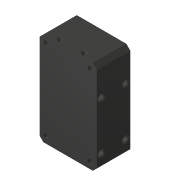
# Autodesk Inventor part: XM430_HOUSING_MIDDLE
Saved by Autodesk Inventor 2019.4 (Build 234330000, 330)
## iProperties
Created: 2019-10-08
Part Number: XM430_HOUSING_MIDDLE
Material: 一般
Document SubType Name: Modeling
Designer: y6tada
Density: 1 g/cm^3
Appearance: 滑らか - 黒
Author: y6tada
Autodesk Inventor part; units mm, degrees
ref_plane "YZ Plane" through (0, 0, 0) normal (1, 0, 0) x (0, 1, 0)
ref_plane "XZ Plane" through (0, 0, 0) normal (0, 1, 0) x (-1, 0, 0)
ref_plane "XY Plane" through (0, 0, 0) normal (0, 0, 1) x (1, 0, 0)
sketch "スケッチ1" plane through (0, 0, 0) normal (0, 0, 1) x (1, 0, 0)
  line L0 (-12.25, 11.25) -> (12.25, 11.25)
  line L1 (14.25, 9.25) -> (14.25, -33.25)
  line L2 (12.25, -35.25) -> (-12.25, -35.25)
  line L3 (-14.25, -33.25) -> (-14.25, 9.25)
  line L4 (0, 0) -> (0, 27.3047) construction
  line L5 (-23.6918, 0) -> (33.2657, 0) construction
  line L6 (-12.25, 11.25) -> (-14.25, 9.25)
  line L7 (12.25, 11.25) -> (14.25, 9.25)
  line L8 (14.25, -33.25) -> (12.25, -35.25)
  line L9 (-12.25, -35.25) -> (-14.25, -33.25)
  circle A0 centre (11, 8) radius 1.25
  circle A1 centre (11, -32) radius 1.25
  line L10 (11, 8) -> (11, -32) construction
  circle A2 centre (-11, 8) radius 1.25
  circle A3 centre (-11, -32) radius 1.25
  point P0 (-14.25, 11.25)
  point P1 (14.25, -35.25)
  point P2 (14.25, 11.25)
  point P3 (-14.25, -35.25)
  dimension "d0" = 11.25
  dimension "d1" = 28.5
  dimension "d2" = 46.5
  dimension "d3" = 2
  dimension "d4" = 2
  dimension "d5" = 2
  dimension "d6" = 2
  dimension "d7" = 2
  dimension "d8" = 2
  dimension "d9" = 2
  dimension "d10" = 2
  dimension "d11" = 22
  dimension "d12" = 8
  dimension "d13" = 40
  dimension "d14" = 2.5
  constraints: 22 end point, 9 point on line, 4 centre point, 2 horizontal, 2 parallel, 2 symmetric about line, 2 vertical, 1 coincident, 1 equal radius, 1 perpendicular, 3 other
  measures "d0" distance between parallel lines of L5 L0
  measures "d1" distance between parallel lines of L1 L3
  measures "d2" distance between parallel lines of L2 L0
  measures "d3" distance of L0.start point (-14.25, 11.25)
  measures "d4" distance of L3.end point (-14.25, 11.25)
  measures "d5" distance of L0.end point (14.25, 11.25)
  measures "d6" distance of L1.start point (14.25, 11.25)
  measures "d7" distance of L1.end point (14.25, -35.25)
  measures "d8" distance of L2.start point (14.25, -35.25)
  measures "d9" distance of L2.end point (-14.25, -35.25)
  measures "d10" distance of L3.start point (-14.25, -35.25)
  measures "d11" diameter of L10 L4
  measures "d12" distance from line of L5 L10.start
  measures "d13" distance of L10.start L10.end
  measures "d14" diameter of A0
extrude "押し出し1" add sketch "スケッチ1" along normal mid plane 16.9
sketch "スケッチ2" plane through (14.25, -33.25, 8.45) normal (1, 0, 0) x (0, 0, -1)
  line L0 (2.45, 29.25) -> (14.45, 29.25) construction
  line L1 (14.45, 29.25) -> (14.45, 5.25) construction
  line L2 (14.45, 5.25) -> (2.45, 5.25) construction
  line L3 (2.45, 5.25) -> (2.45, 29.25) construction
  line L4 (8.45, 45.5456) -> (8.45, -6.7965) construction
  line L5 (-14.7674, 33.25) -> (26.9277, 33.25) construction
  circle A0 centre (2.45, 29.25) radius 1.25
  circle A1 centre (14.45, 29.25) radius 1.25
  circle A2 centre (14.45, 5.25) radius 1.25
  circle A3 centre (2.45, 5.25) radius 1.25
  point P0 (8.45, 33.25)
  dimension "d17" = 12
  dimension "d18" = 4
  dimension "d19" = 24
  dimension "d20" = 2.5
  constraints: 12 end point, 4 centre point, 4 coincident, 3 equal radius, 2 horizontal, 2 parallel, 2 point on line, 1 perpendicular, 1 vertical, 1 other
  measures "d17" distance of L0.start L0.end
  measures "d18" distance from line of L0 point (8.45, 33.25)
  measures "d19" distance between parallel lines of L2 L0
  measures "d20" diameter of A1
extrude "押し出し2" cut sketch "スケッチ2" against normal blind 3
mirror "ミラー1" about plane through (0, 0, 0) normal (1, 0, 0) of "押し出し2"
sketch "スケッチ3" plane through (-12.25, 11.25, 8.45) normal (0, 1, 0) x (1, 0, 0)
  line L0 (12.25, 8.45) -> (12.25, -3.712) construction
  line L1 (6.25, 2.45) -> (18.25, 2.45) construction
  circle A0 centre (6.25, 2.45) radius 1.25
  circle A1 centre (18.25, 2.45) radius 1.25
  dimension "d23" = 2.5
  dimension "d24" = 12
  dimension "d25" = 6
  constraints: 4 end point, 2 centre point, 2 coincident, 1 equal radius, 1 horizontal, 1 symmetric about line, 1 vertical
  measures "d23" diameter of A0
  measures "d24" distance of L1.start L1.end
  measures "d25" distance from line of L0.start L1
extrude "押し出し3" cut sketch "スケッチ3" against normal blind 3
sketch "スケッチ4" plane through (-12.25, -35.25, 8.45) normal (0, -1, 0) x (1, 0, 0)
  line L0 (12.25, 3.9965) -> (12.25, -24.0528) construction
  line L1 (4.25, -2.45) -> (20.25, -2.45) construction
  line L2 (20.25, -2.45) -> (20.25, -14.45) construction
  line L3 (20.25, -14.45) -> (4.25, -14.45) construction
  line L4 (4.25, -14.45) -> (4.25, -2.45) construction
  circle A0 centre (4.25, -2.45) radius 1.25
  circle A1 centre (4.25, -14.45) radius 1.25
  circle A2 centre (20.25, -2.45) radius 1.25
  circle A3 centre (20.25, -14.45) radius 1.25
  line L5 (-5.6157, -8.45) -> (30.9537, -8.45) construction
  point P0 (12.25, -8.45)
  dimension "d64" = 12
  dimension "d65" = 16
  dimension "d66" = 2.5
  constraints: 12 end point, 4 centre point, 4 coincident, 3 equal radius, 2 horizontal, 2 parallel, 2 point on line, 1 perpendicular, 1 vertical, 2 other
  measures "d64" distance of L1.end L2.end
  measures "d65" distance of L1.start L1.end
  measures "d66" diameter of A2
extrude "押し出し4" cut sketch "スケッチ4" against normal blind 3
chamfer "面取り1" distance 0.2 angle 45 16 edges at (-14.25, -12, 8.45) (-13.25, -34.25, 8.45) (0, -35.25, 8.45) (13.25, -34.25, 8.45) (14.25, -12, 8.45) (13.25, 10.25, 8.45) (0, 11.25, 8.45) (-13.25, 10.25, 8.45) (13.25, 10.25, -8.45) (0, 11.25, -8.45) (-13.25, 10.25, -8.45) (-14.25, -12, -8.45) (-13.25, -34.25, -8.45) (0, -35.25, -8.45) (13.25, -34.25, -8.45) (14.25, -12, -8.45)
chamfer "面取り2" distance 0.35 angle 45 14 edges at (-14.25, -4, 7.25) (-14.25, -4, -4.75) (-14.25, -28, -4.75) (-14.25, -28, 7.25) (-7.25, 11.25, 6) (4.75, 11.25, 6) (14.25, -4, 7.25) (14.25, -4, -4.75) (14.25, -28, -4.75) (14.25, -28, 7.25) (6.75, -35.25, 6) (-9.25, -35.25, 6) (-9.25, -35.25, -6) (6.75, -35.25, -6)
sketch "スケッチ5" plane through (0, 0, -8.45) normal (0, 0, -1) x (-1, 0, 0)
  line L0 (12.25, 11.25) -> (-12.25, 11.25) construction
  line L1 (14.25, -33.25) -> (14.25, 9.25) construction
  circle A0 centre (11, 8) radius 1.25 construction
  line L2 (8, 10.05) -> (-8, 10.05)
  line L3 (13.05, -25.25) -> (13.05, -6.75)
  line L4 (0, -4) -> (14.25, -4) construction
  line L5 (12.05, -2.25) -> (10.75, -2.25)
  line L6 (10.45, -2.55) -> (10.45, -5.45)
  line L7 (10.75, -5.75) -> (12.05, -5.75)
  line L8 (13.05, -1.25) -> (13.05, 5)
  line L9 (13.05, -5.75) -> (13.05, -2.25) construction
  arc A1 (9, 8) -> (11, 6) centre (11, 8) ccw
  line L10 (9, 9.05) -> (9, 8)
  line L11 (11, 6) -> (12.05, 6)
  line L12 (-12.25, -35.25) -> (12.25, -35.25) construction
  line L13 (0, -12) -> (14.25, -12) construction
  line L14 (8, -35.25) -> (8, -32.724) construction
  line L15 (8.2728, -31.75) -> (6.8, -31.75)
  line L16 (6.3, -32.25) -> (6.3, -33.05)
  line L17 (5.3, -34.05) -> (-5.3, -34.05)
  line L18 (-12.25, 11.25) -> (12.25, 11.25) construction
  line L19 (0, 11.25) -> (0, -35.25) construction
  line L20 (10.45, -29.4314) -> (10.45, -26.75)
  line L21 (10.95, -26.25) -> (12.05, -26.25)
  line L22 (10.45, -28) -> (14.25, -28) construction
  arc A2 (9.9667, -30.2876) -> (9.1819, -31.1667) centre (11, -32) ccw
  circle A3 centre (11, -32) radius 1.25 construction
  arc A4 (5.3, -34.05) -> (6.3, -33.05) centre (5.3, -33.05) ccw
  arc A5 (8.2728, -31.75) -> (9.1819, -31.1667) centre (8.2728, -30.75) ccw
  arc A6 (9.9667, -30.2876) -> (10.45, -29.4314) centre (9.45, -29.4314) ccw
  arc A7 (12.05, -26.25) -> (13.05, -25.25) centre (12.05, -25.25) ccw
  arc A8 (13.05, -6.75) -> (12.05, -5.75) centre (12.05, -6.75) ccw
  arc A9 (12.05, -2.25) -> (13.05, -1.25) centre (12.05, -1.25) ccw
  arc A10 (13.05, 5) -> (12.05, 6) centre (12.05, 5) ccw
  arc A11 (9, 9.05) -> (8, 10.05) centre (8, 9.05) ccw
  line L23 (6.3, -32.25) -> (6.8, -31.75)
  line L24 (10.45, -26.75) -> (10.95, -26.25)
  arc A12 (10.45, -5.45) -> (10.75, -5.75) centre (10.75, -5.45) ccw
  arc A13 (10.75, -2.25) -> (10.45, -2.55) centre (10.75, -2.55) ccw
  line L25 (-14.25, -33.25) -> (-14.25, 9.25) construction
  circle A14 centre (-11, 8) radius 1.25 construction
  line L26 (-13.05, -25.25) -> (-13.05, -6.75)
  line L27 (-12.05, -2.25) -> (-10.75, -2.25)
  line L28 (-10.45, -2.55) -> (-10.45, -5.45)
  line L29 (-10.75, -5.75) -> (-12.05, -5.75)
  line L30 (-13.05, -1.25) -> (-13.05, 5)
  line L31 (-13.05, -5.75) -> (-13.05, -2.25) construction
  arc A15 (-11, 6) -> (-9, 8) centre (-11, 8) ccw
  line L32 (-9, 9.05) -> (-9, 8)
  line L33 (-11, 6) -> (-12.05, 6)
  line L34 (-8, -35.25) -> (-8, -32.724) construction
  line L35 (-8.2728, -31.75) -> (-6.8, -31.75)
  line L36 (-6.3, -32.25) -> (-6.3, -33.05)
  line L37 (-10.45, -29.4314) -> (-10.45, -26.75)
  line L38 (-10.95, -26.25) -> (-12.05, -26.25)
  line L39 (-10.45, -28) -> (-14.25, -28) construction
  arc A16 (-9.1819, -31.1667) -> (-9.9667, -30.2876) centre (-11, -32) ccw
  circle A17 centre (-11, -32) radius 1.25 construction
  arc A18 (-6.3, -33.05) -> (-5.3, -34.05) centre (-5.3, -33.05) ccw
  arc A19 (-9.1819, -31.1667) -> (-8.2728, -31.75) centre (-8.2728, -30.75) ccw
  arc A20 (-10.45, -29.4314) -> (-9.9667, -30.2876) centre (-9.45, -29.4314) ccw
  arc A21 (-13.05, -25.25) -> (-12.05, -26.25) centre (-12.05, -25.25) ccw
  arc A22 (-12.05, -5.75) -> (-13.05, -6.75) centre (-12.05, -6.75) ccw
  arc A23 (-13.05, -1.25) -> (-12.05, -2.25) centre (-12.05, -1.25) ccw
  arc A24 (-12.05, 6) -> (-13.05, 5) centre (-12.05, 5) ccw
  arc A25 (-8, 10.05) -> (-9, 9.05) centre (-8, 9.05) ccw
  line L40 (-6.3, -32.25) -> (-6.8, -31.75)
  line L41 (-10.45, -26.75) -> (-10.95, -26.25)
  arc A26 (-10.75, -5.75) -> (-10.45, -5.45) centre (-10.75, -5.45) ccw
  arc A27 (-10.45, -2.55) -> (-10.75, -2.25) centre (-10.75, -2.55) ccw
  point P0 (0, 0)
  point P1 (6.3, -31.75)
  point P2 (10.45, -26.25)
  point P3 (10.45, -30.0771)
  point P4 (9.0157, -31.75)
  point P5 (-6.3, -31.75)
  point P6 (-10.45, -26.25)
  point P7 (-10.45, -30.0771)
  point P8 (-9.0157, -31.75)
  dimension "d37" = 4
  dimension "d38" = 1.2
  dimension "d39" = 1.2
  dimension "d41" = 2
  dimension "d42" = 3.8
  dimension "d43" = 3.5
  dimension "d44" = 8
  dimension "d45" = 3.4
  dimension "d46" = 3.5
  dimension "d47" = 1.2
  dimension "d48" = 3.5
  dimension "d49" = 24
  dimension "d50" = 2
  dimension "d51" = 1
  dimension "d52" = 0.5
  dimension "d53" = 0.5
  dimension "d54" = 0.5
  dimension "d55" = 0.5
  dimension "d56" = 0.3
  constraints: 76 end point, 52 point on circle, 52 symmetric about line, 27 point on line, 26 centre point, 22 tangent, 13 perpendicular, 8 equal radius, 4 horizontal, 4 midpoint, 4 parallel, 2 coincident, 2 vertical, 1 collinear, 1 concentric, 15 other
  measures "d37" distance from line of L4 point (0, 0)
  measures "d38" distance between parallel lines of L1 L8
  measures "d39" distance between parallel lines of L2 L0
  measures "d41" radius of A1
  measures "d42" distance between parallel lines of L1 L6
  measures "d43" distance between parallel lines of L7 L5
  measures "d44" distance between parallel lines of L19 L14
  measures "d45" diameter of L16 L14
  measures "d46" distance between parallel lines of L12 L15
  measures "d47" distance between parallel lines of L12 L17
  measures "d48" diameter of L21 L22
  measures "d49" distance between parallel lines of L4 L22
  measures "d50" radius of A2
  measures "d51" radius of A4
  measures "d52" distance of L16.start point (6.3, -31.75)
  measures "d53" distance of L15.end point (6.3, -31.75)
  measures "d54" distance of L20.end point (10.45, -26.25)
  measures "d55" distance of L21.start point (10.45, -26.25)
  measures "d56" radius of A12
extrude "押し出し5" cut sketch "スケッチ5" against normal blind 12.35
sketch "スケッチ7" plane through (0, 0, -8.45) normal (0, 0, -1) x (-1, 0, 0)
  line L0 (12.25, 11.25) -> (-12.25, 11.25) construction
  line L1 (14.25, 9.25) -> (12.25, 11.25) construction
  line L2 (14.25, -33.25) -> (14.25, 9.25) construction
  line L3 (12.25, -35.25) -> (14.25, -33.25) construction
  line L4 (-12.25, -35.25) -> (12.25, -35.25) construction
  line L5 (-14.25, -33.25) -> (-12.25, -35.25) construction
  line L6 (-14.25, 9.25) -> (-14.25, -33.25) construction
  line L7 (-12.25, 11.25) -> (-14.25, 9.25) construction
  line L8 (-11.9932, 10.63) -> (11.9932, 10.63)
  line L9 (11.9932, 10.63) -> (13.63, 8.9932)
  line L10 (13.63, 8.9932) -> (13.63, -32.9932)
  line L11 (13.63, -32.9932) -> (11.9932, -34.63)
  line L12 (11.9932, -34.63) -> (-11.9932, -34.63)
  line L13 (-11.9932, -34.63) -> (-13.63, -32.9932)
  line L14 (-13.63, -32.9932) -> (-13.63, 8.9932)
  line L15 (-13.63, 8.9932) -> (-11.9932, 10.63)
  point P0 (0, 0)
  dimension "d67" = 0.62
  constraints: 16 end point, 7 other
  measures "d67" distance between parallel lines of L0 L8
extrude "押し出し7" cut sketch "スケッチ7" against normal blind 0.75
sketch "スケッチ6" plane through (0, 0, 3.9) normal (0, 0, -1) x (-1, 0, 0)
  circle A0 centre (1.21, -25.01) radius 8.7
  line L0 (-12.25, -35.25) -> (12.25, -35.25) construction
  line L1 (14.25, -33.25) -> (14.25, 9.25) construction
  line L2 (-12.25, -33.71) -> (12.25, -33.71) construction
  line L3 (9.91, -33.25) -> (9.91, 9.25) construction
  point P0 (0, 0)
  dimension "d59" = 17.4
  dimension "d60" = 4.34
  dimension "d61" = 1.54
  constraints: 4 end point, 2 parallel, 2 tangent, 1 centre point
  measures "d59" diameter of A0
  measures "d60" distance between parallel lines of L1 L3
  measures "d61" distance between parallel lines of L0 L2
extrude "押し出し6" add sketch "スケッチ6" along normal blind 17.48
equation "\"d4\" = d3"
equation "\"d5\" = d3"
equation "\"d6\" = d5"
equation "\"d7\" = d3"
equation "\"d8\" = d7"
equation "\"d9\" = d3"
equation "\"d10\" = d9"
equation "\"d53\" = d52"
equation "\"d54\" = d52"
equation "\"d55\" = d54"
